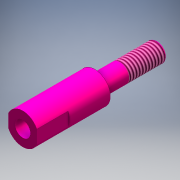
# Autodesk Inventor part: Semi albero F
Saved by Autodesk Inventor 2016 (Build 200138000, 138)
## iProperties
Created: 2016-09-10
Part Number: Semi albero F
Material: Generic
Document SubType Name: Modeling
Designer: Muhammad
Density: 1 g/cm^3
Appearance: Default
Author: Muhammad
Autodesk Inventor part; units mm, degrees
ref_plane "YZ Plane" through (0, 0, 0) normal (1, 0, 0) x (0, 1, 0)
ref_plane "XZ Plane" through (0, 0, 0) normal (0, 1, 0) x (-1, 0, 0)
ref_plane "XY Plane" through (0, 0, 0) normal (0, 0, 1) x (1, 0, 0)
sketch "Sketch1" plane through (0, 0, 0) normal (0, 1, 0) x (-1, 0, 0)
  circle A0 centre (0, 0) radius 5
  dimension "d0" = 10
  constraints: 1 centre point, 1 coincident
  measures "d0" diameter of A0
extrude "Extrusion1" add sketch "Sketch1" along normal blind 23
sketch "Sketch2" plane through (0, 23, 0) normal (0, 1, 0) x (1, 0, 0)
  circle A0 centre (0, 0) radius 3
  dimension "d3" = 6
  constraints: 1 centre point, 1 coincident
  measures "d3" diameter of A0
extrude "Extrusion2" add sketch "Sketch2" along normal blind 20
thread "Thread1" size "M6x1" class "6g" standard "ANSI Metric M Profile" length 12
fillet "Fillet1" radius 0.5 1 edges at (-3, 43, 0)
sketch "Sketch3" plane through (0, 0, 0) normal (0, -1, 0) x (1, 0, 0)
  line L0 (4.5, 0) -> (-4.5, 0) construction
  circle A0 centre (0, 0) radius 5 projected
  line L1 (4.5, -2.1794) -> (4.5, 2.1794)
  line L2 (-4.5, -2.1794) -> (-4.5, 2.1794)
  constraints: 6 end point, 4 point on circle, 1 perpendicular, 1 vertical
extrude "Extrusion3" cut sketch "Sketch3" against normal blind 10 contours A0 L1 | L2 A0
sketch "Sketch4" plane through (0, 0, 0) normal (0, -1, 0) x (1, 0, 0)
  line L0 (3.705, 0) -> (-3.8794, 0) construction
  point P0 (0, 0)
  constraints: 2 end point, 1 horizontal
hole "Hole1" at (0, 0, 0) direction (0, 1, 0) diameter 5 depth 14 tip angle 118
body "Solid1"
